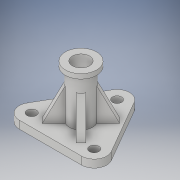
# Autodesk Inventor part: 練習二
Saved by Autodesk Inventor 2017 (Build 210142000, 142)
## iProperties
Part Number: 練習二
Material: 一般
Document SubType Name: Modeling
Designer: user
Density: 1 g/cm^3
Appearance: 預設
Author: user
Autodesk Inventor part; units mm, degrees
ref_plane "XZ Plane" through (0, 0, 0) normal (0, 1, 0) x (-1, 0, 0)
ref_plane "XY Plane" through (0, 0, 0) normal (0, 0, 1) x (1, 0, 0)
sketch "草圖1" plane through (0, 0, 0) normal (0, 1, 0) x (-1, 0, 0)
  line L0 (-13.8564, -54.188) -> (-53.8564, 15.094)
  line L1 (-40, 39.094) -> (40, 39.094)
  line L2 (53.8564, 15.094) -> (13.8564, -54.188)
  arc A0 (-13.8564, -54.188) -> (13.8564, -54.188) centre (0, -46.188) ccw
  arc A1 (-40, 39.094) -> (-53.8564, 15.094) centre (-40, 23.094) ccw
  arc A2 (53.8564, 15.094) -> (40, 39.094) centre (40, 23.094) ccw
  line L3 (0, 0) -> (0, 68.1161)
  point P0 (0, -78.188)
  point P1 (-67.7128, 39.094)
  point P2 (67.7128, 39.094)
  dimension "d0" = 16
  dimension "d1" = 80
  dimension "d2" = 90
  constraints: 8 end point, 6 point on circle, 6 point on line, 6 tangent, 3 centre point, 2 equal radius, 1 coincident, 1 vertical, 7 other
  measures "d0" radius of A0
  measures "d1" distance of A1.centre A2.centre
  measures "d2" angle of L3 L1
extrude "擠出1" add sketch "草圖1" along normal blind 10
sketch "草圖3" plane through (0, 10, 0) normal (0, 1, 0) x (1, 0, 0)
  line L0 (-40, -39.094) -> (40, -39.094) projected
  line L1 (0, -39.094) -> (0, 73.5)
  line L2 (53.8564, -15.094) -> (13.8564, 54.188) projected
  line L3 (33.8564, 19.547) -> (-74.1911, -42.8343)
  line L4 (-13.8564, 54.188) -> (-53.8564, -15.094) projected
  line L5 (-33.8564, 19.547) -> (58.7695, -33.9306)
  circle A0 centre (0, 0) radius 15
  dimension "d11" = 30
  constraints: 6 end point, 3 midpoint, 2 perpendicular, 1 centre point, 1 coincident, 1 vertical
  measures "d11" diameter of A0
extrude "擠出3" add sketch "草圖3" along normal blind 60
sketch "草圖4" plane through (0, 70, 0) normal (0, 1, 0) x (1, 0, 0)
  circle A0 centre (0, 0) radius 20
  dimension "d14" = 40
  constraints: 1 centre point, 1 coincident
  measures "d14" diameter of A0
extrude "擠出4" add sketch "草圖4" along normal blind 6
sketch "草圖5" plane through (0, 76, 0) normal (0, 1, 0) x (1, 0, 0)
  circle A0 centre (0, 0) radius 11
  dimension "d17" = 22
  constraints: 1 centre point, 1 coincident
  measures "d17" diameter of A0
extrude "擠出5" cut sketch "草圖5" against normal up to next
sketch "草圖6" plane through (0, 10, 0) normal (0, 1, 0) x (1, 0, 0)
  arc A0 (13.8564, 54.188) -> (-13.8564, 54.188) centre (0, 46.188) ccw projected
  circle A1 centre (0, 46.188) radius 6
  arc A2 (-53.8564, -15.094) -> (-40, -39.094) centre (-40, -23.094) ccw projected
  circle A3 centre (-40, -23.094) radius 6
  arc A4 (40, -39.094) -> (53.8564, -15.094) centre (40, -23.094) ccw projected
  circle A5 centre (40, -23.094) radius 6
  point P0 (0, 0)
  dimension "d20" = 12
  dimension "d21" = 12
  dimension "d22" = 12
  constraints: 3 centre point, 3 coincident
  measures "d20" diameter of A3
  measures "d21" diameter of A1
  measures "d22" diameter of A5
extrude "擠出6" cut sketch "草圖6" against normal up to next
ref_plane "工作平面2" through (0, 76, 0) normal (0.7071068, 0, -0.7071068) x (0, 1, 0)
ref_plane "工作平面3" through (0, 76, 0) normal (0.7071068, 0, -0.7071068) x (0, 1, 0)
ref_plane "工作平面4" through (0, 76, 0) normal (0, 0, -1) x (0, 1, 0)
sketch "草圖9" plane through (0, 76, 0) normal (0.7071068, 0, -0.7071068) x (0, 1, 0)
  line L0 (-66, 15) -> (-6, 15) projected
  line L1 (-26, 15) -> (-66, 35)
  line L2 (-66, -0.6406) -> (-66, 55.9279) projected
  point P0 (-76, 0)
  dimension "d30" = 40
  dimension "d31" = 20
  constraints: 2 end point, 2 point on line
  measures "d30" distance from line of L2 L1.start
  measures "d31" distance from line of L1.end L0
extrude "肋1" add sketch "草圖9" along normal mid plane 9 rib yes fills toward (-46.0224, 24.9553) open curves L1
pattern_circular "環形陣列1" count 4 over 360 about axis through (0, 76, 0) along (0, 1, 0) of "肋1"
